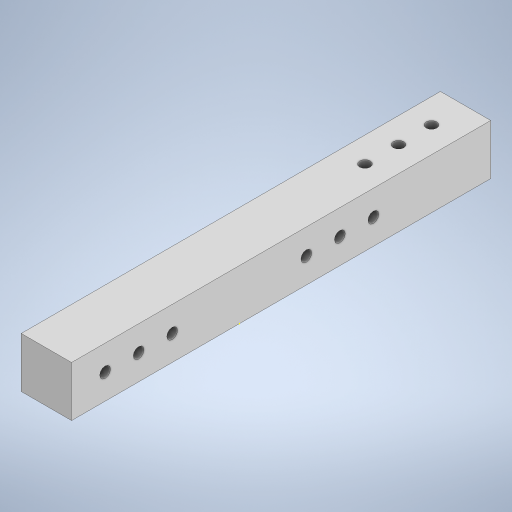
# Autodesk Inventor part: 射出_角柱10
Saved by Autodesk Inventor 2023 (Build 270158000, 158)
## iProperties
Created: 2022-04-19
Part Number: 射出_角柱10
Material: 一般
Document SubType Name: Modeling
Designer: yuta
Density: 1 g/cm^3
Appearance: 既定
Author: yuta
Autodesk Inventor part; units mm, degrees
ref_plane "YZ Plane" through (0, 0, 0) normal (1, 0, 0) x (0, 1, 0)
ref_plane "XZ Plane" through (0, 0, 0) normal (0, 1, 0) x (-1, 0, 0)
ref_plane "XY Plane" through (0, 0, 0) normal (0, 0, 1) x (1, 0, 0)
sketch "スケッチ1" plane through (0, 0, 0) normal (0, 0, 1) x (1, 0, 0)
  line L0 (0, 0) -> (15, 0)
  line L1 (15, 0) -> (15, 15)
  line L2 (15, 15) -> (0, 15)
  line L3 (0, 15) -> (0, 0)
  dimension "d0" = 15
  dimension "d1" = 15
  constraints: 8 end point, 2 parallel, 1 horizontal, 1 perpendicular
  measures "d0" distance of L2.end L1.end
  measures "d1" distance of L1.end L0.end
extrude "押し出し1" add sketch "スケッチ1" along normal blind 50
sketch "スケッチ3" plane through (0, 0, 0) normal (0, 0, -1) x (-1, 0, 0)
  line L0 (0, 15) -> (0, 0) projected
  line L1 (0, 0) -> (-15, 0)
  line L2 (-15, 0) -> (-15, 15)
  line L3 (-15, 15) -> (0, 15)
  line L4 (0, 15) -> (0, 0)
  dimension "d21" = 15
  dimension "d22" = 15
  constraints: 8 end point, 2 parallel, 1 horizontal, 1 perpendicular
  measures "d21" distance of L2.end L3.end
  measures "d22" distance of L1.end L2.end
extrude "押し出し2" add sketch "スケッチ3" along normal blind 135
sketch "スケッチ4" plane through (0, 15, 50) normal (0, 1, 0) x (1, 0, 0)
  line L0 (15, 0) -> (15, 185) projected
  line L1 (15, 185) -> (0, 185)
  line L2 (0, 185) -> (0, 105)
  line L3 (0, 105) -> (15, 105)
  line L4 (15, 105) -> (15, 185)
  point P0 (0, 50)
  dimension "d25" = 15
  dimension "d26" = 80
  constraints: 8 end point, 2 parallel, 1 horizontal, 1 perpendicular
  measures "d25" distance of L3.end L2.end
  measures "d26" distance of L2.end L1.end
extrude "押し出し3" cut sketch "スケッチ4" against normal blind 135
sketch "スケッチ5" plane through (15, 15, -55) normal (0, 0, -1) x (-1, 0, 0)
  line L0 (15, 0) -> (15, -15) projected
  line L1 (0, -15) -> (0, 0) projected
  line L2 (15, -15) -> (0, -15)
  line L3 (0, -15) -> (0, 0)
  line L4 (0, 0) -> (15, 0)
  line L5 (15, 0) -> (15, -15)
  constraints: 8 end point, 2 parallel, 1 horizontal, 1 perpendicular
extrude "押し出し4" add sketch "スケッチ5" along normal blind 15
sketch "スケッチ8" plane through (15, 0, 50) normal (1, 0, 0) x (0, 0, -1)
  line L0 (120, 15) -> (120, 0) projected
  line L1 (120, 15) -> (0, 15) projected
  point P0 (50, 0)
  point P1 (90, 7.5)
  point P2 (80, 7.5)
  point P3 (70, 7.5)
  dimension "d54" = 30
  dimension "d55" = 7.5
  dimension "d56" = 7.5
  dimension "d57" = 7.5
  dimension "d58" = 10
  dimension "d59" = 10
  measures "d54" distance from line of L0 point (90, 7.5)
  measures "d55" distance from line of L1 point (90, 7.5)
  measures "d56" distance from line of L1 point (70, 7.5)
  measures "d57" distance from line of L1 point (80, 7.5)
  measures "d58" distance of point (90, 7.5) point (80, 7.5)
  measures "d59" distance of point (80, 7.5) point (70, 7.5)
hole "穴4" at (15, 7.5, -40) at (15, 7.5, -30) at (15, 7.5, -20) direction (-1, 0, 0) diameter 3.2 end through all
sketch "スケッチ9" plane through (15, 0, 50) normal (1, 0, 0) x (0, 0, -1)
  line L0 (0, 0) -> (0, 15) projected
  line L1 (0, 0) -> (120, 0) projected
  point P0 (50, 0)
  point P1 (10, 7.5)
  point P2 (20, 7.5)
  dimension "d67" = 10
  dimension "d68" = 10
  dimension "d69" = 7.5
  dimension "d70" = 7.5
  measures "d67" distance from line of L0 point (10, 7.5)
  measures "d68" distance of point (10, 7.5) point (20, 7.5)
  measures "d69" distance from line of L1 point (10, 7.5)
  measures "d70" distance from line of L1 point (20, 7.5)
hole "穴5" at (15, 7.5, 40) at (15, 7.5, 30) direction (-1, 0, 0) diameter 3.2 end through all
sketch "スケッチ10" plane through (15, 0, 50) normal (1, 0, 0) x (0, 0, -1)
  point P0 (50, 0)
sketch "スケッチ11" plane through (15, 0, 50) normal (1, 0, 0) x (0, 0, -1)
  line L0 (0, 0) -> (0, 15) projected
  line L1 (0, 0) -> (120, 0) projected
  point P0 (50, 0)
  point P1 (30, 7.5)
  dimension "d78" = 30
  dimension "d79" = 7.5
  measures "d78" distance from line of L0 point (30, 7.5)
  measures "d79" distance from line of L1 point (30, 7.5)
hole "穴6" at (15, 7.5, 20) direction (-1, 0, 0) diameter 3.2 end through all
sketch "スケッチ12" plane through (15, 15, -70) normal (0, 0, -1) x (-1, 0, 0)
  line L0 (0, 0) -> (0, -15) projected
  line L1 (0, 0) -> (15, 0)
  line L2 (15, 0) -> (15, -15)
  line L3 (15, -15) -> (0, -15)
  line L4 (0, -15) -> (0, 0)
  constraints: 8 end point, 2 parallel, 1 horizontal, 1 perpendicular
extrude "押し出し5" add sketch "スケッチ12" along normal blind 5
sketch "スケッチ13" plane through (0, 15, 50) normal (0, 1, 0) x (1, 0, 0)
  line L0 (0, 125) -> (15, 125) projected
  point P0 (0, 50)
  point P1 (7.3304, 115)
  point P2 (7.5, 105)
  point P3 (7.5, 95)
  dimension "d89" = 10
  dimension "d90" = 10
  dimension "d91" = 10
  measures "d89" distance from line of L0 point (7.33, 115)
  measures "d90" vertical distance of point (7.5, 105) point (7.33, 115)
  measures "d91" distance of point (7.5, 95) point (7.5, 105)
hole "穴7" at (7.5, 15, -45) at (7.5, 15, -55) at (7.3304, 15, -65) direction (0, -1, 0) diameter 3.2 end through all
